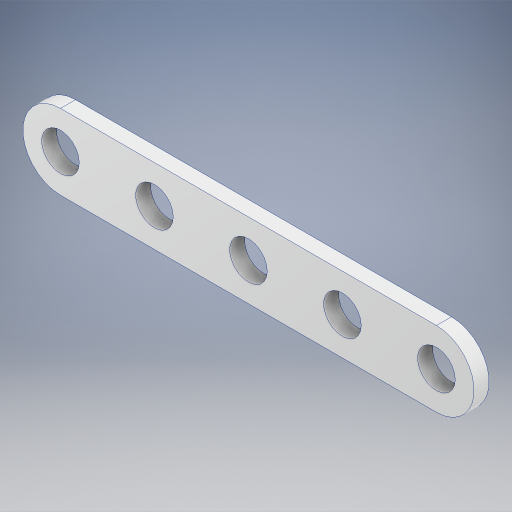
# Autodesk Inventor part: CE-10.2.1
Saved by Autodesk Inventor 2024 (Build 280153000, 153)
## iProperties
Created: 2024-03-22
Part Number: CE-10.2.1
Material: Aluminum 6061
Document SubType Name: Modeling
Designer: Alex
Density: 2.7 g/cm^3
Appearance: Aluminum - Flat
Author: Alex
Autodesk Inventor part; units mm, degrees
ref_plane "YZ Plane" through (0, 0, 0) normal (1, 0, 0) x (0, 1, 0)
ref_plane "XZ Plane" through (0, 0, 0) normal (0, 1, 0) x (-1, 0, 0)
ref_plane "XY Plane" through (0, 0, 0) normal (0, 0, 1) x (1, 0, 0)
sketch "Sketch1" plane through (0, 0, 0) normal (0, 0, 1) x (1, 0, 0)
  line L0 (-250, 0) -> (250, 0) construction
  line L1 (-250, -50) -> (250, -50)
  line L2 (250, 50) -> (-250, 50)
  arc A0 (-250, 50) -> (-250, -50) centre (-250, 0) ccw
  arc A1 (250, -50) -> (250, 50) centre (250, 0) ccw
  circle A2 centre (-250, 0) radius 25
  circle A3 centre (0, 0) radius 25
  circle A4 centre (250, 0) radius 25
  circle A5 centre (-125, 0) radius 25
  circle A6 centre (125, 0) radius 25
  dimension "d0" = 500
  dimension "d1" = 50
  dimension "d2" = 50
  dimension "d3" = 125
  dimension "d4" = 125
  constraints: 8 end point, 7 centre point, 4 equal radius, 4 point on circle, 4 tangent, 3 coincident, 2 point on line, 1 horizontal, 1 midpoint, 1 parallel
  measures "d0" distance of L2.start L2.end
  measures "d1" radius of A1
  measures "d2" diameter of A2
  measures "d3" distance of A5.centre L0.start
  measures "d4" distance of A6.centre point (0, 0)
extrude "Extrusion1" add sketch "Sketch1" along normal mid plane 20
body "Solid1"
